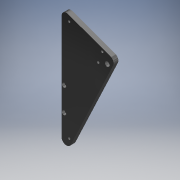
# Autodesk Inventor part: Triangle axle slide connector
Saved by Autodesk Inventor 2019 (Build 230136000, 136)
## iProperties
Part Number: Triangle axle slide connector
Material: Generic
Document SubType Name: Modeling
Designer: Delta
Appearance: Default
Author: Delta
Autodesk Inventor part; units mm, degrees
ref_plane "YZ Plane" through (0, 0, 0) normal (1, 0, 0) x (0, 1, 0)
ref_plane "XZ Plane" through (0, 0, 0) normal (0, 1, 0) x (-1, 0, 0)
ref_plane "XY Plane" through (0, 0, 0) normal (0, 0, 1) x (1, 0, 0)
sketch "Sketch1" plane through (0, 0, 0) normal (0, 0, 1) x (1, 0, 0)
  line L0 (0, 0) -> (0, 177.8)
  line L1 (0, 0) -> (53.8815, 0) construction
  line L2 (0, 177.8) -> (71.6046, 151.7381)
  line L3 (0, 177.8) -> (76.2, 177.8) construction
  line L4 (71.6046, 151.7381) -> (0, 0)
  dimension "d0" = 177.8
  dimension "d19" = 76.2
  dimension "d20" = 20
  constraints: 10 end point, 2 horizontal, 1 equal length, 1 vertical
  measures "d0" distance of L0.start L0.end
  measures "d19" distance of L0.end L2.end
  measures "d20" angle of L2 L3
extrude "Extrusion1" add sketch "Sketch1" along normal blind 6.35
fillet "Fillet1" radius 6.35 2 edges at (0, 177.8, 3.175) (0, 0, 3.175)
fillet "Fillet4" radius 6.35 1 edges at (71.6046, 151.7381, 3.175)
sketch "Sketch3" plane through (0, 0, 6.35) normal (0, 0, 1) x (1, 0, 0)
  circle A0 centre (3.175, 58.1807) radius 1.524
  circle A1 centre (3.175, 89.9307) radius 1.524
  line L0 (0, 168.7313) -> (0, 28.3357) projected
  point P0 (0, 0)
  dimension "d22" = 3.048
  dimension "d23" = 3.048
  dimension "d24" = 3.175
  dimension "d25" = 3.175
  dimension "d26" = 29.845
  dimension "d27" = 31.75
  constraints: 2 centre point
  measures "d22" diameter of A0
  measures "d23" diameter of A1
  measures "d24" distance from line of L0 A0.centre
  measures "d25" distance from line of L0 A1.centre
  measures "d26" vertical distance of L0.end A0.centre
  measures "d27" distance of A0.centre A1.centre
extrude "Extrusion3" cut sketch "Sketch3" against normal through all
sketch "Sketch4" plane through (0, 0, 6.35) normal (0, 0, 1) x (1, 0, 0)
  circle A0 centre (3.175, 58.1807) radius 1.524 projected
  circle A1 centre (3.175, 58.1807) radius 2.921
  circle A2 centre (3.175, 89.9307) radius 1.524 projected
  circle A3 centre (3.175, 89.9307) radius 2.921
  point P0 (0, 0)
  dimension "d30" = 5.842
  dimension "d31" = 5.842
  constraints: 2 centre point, 2 coincident
  measures "d30" diameter of A1
  measures "d31" diameter of A3
extrude "Extrusion4" cut sketch "Sketch4" against normal blind 3.556
sketch "Sketch5" plane through (0, 0, 6.35) normal (0, 0, 1) x (1, 0, 0)
  circle A0 centre (60.795, 143.1007) radius 3.175
  point P0 (0, 0)
  point P1 (8.5218, 174.6983)
  dimension "d34" = 6.35
  dimension "d35" = 52.2732
  dimension "d36" = 31.5976
  constraints: 1 centre point
  measures "d34" diameter of A0
  measures "d35" horizontal distance of point (8.522, 174.698) A0.centre
  measures "d36" vertical distance of A0.centre point (8.522, 174.698)
extrude "Extrusion5" cut sketch "Sketch5" against normal through all
sketch "Sketch6" plane through (0, 0, 6.35) normal (0, 0, 1) x (1, 0, 0)
  line L0 (0, 168.7313) -> (0, 28.3357) projected
  arc A0 (8.5218, 174.6983) -> (0, 168.7313) centre (6.35, 168.7313) ccw projected
  point P0 (0, 0)
  point P1 (10.0076, 166.8263)
  point P2 (10.0076, 31.8253)
  dimension "d39" = 10.0076
  dimension "d40" = 1.905
  dimension "d41" = 136.906
  dimension "d42" = 0
  measures "d39" distance from line of L0 point (10.008, 166.826)
  measures "d40" vertical distance of A0.centre point (10.008, 166.826)
  measures "d41" vertical distance of point (10.008, 31.825) A0.centre
  measures "d42" horizontal distance of point (10.008, 31.825) point (10.008, 166.826)
hole "Hole1" at (10.0076, 31.8253, 6.35) at (10.0076, 166.8263, 6.35) direction (0, 0, -1) diameter 3 end through all
sketch "Sketch7" plane through (0, 0, 6.35) normal (0, 0, 1) x (1, 0, 0)
  line L0 (65.0627, 154.1191) -> (8.5218, 174.6983) projected
  line L1 (12.0927, 25.6258) -> (68.6335, 145.4421) projected
  circle A0 centre (48.6603, 139.0056) radius 1.5875
  circle A1 centre (54.0562, 154.0707) radius 1.5875
  point P0 (0, 0)
  dimension "d52" = 3.81
  dimension "d53" = 19.812
  dimension "d54" = 15.3162
  dimension "d55" = 16.8656
  dimension "d56" = 3.175
  dimension "d57" = 3.175
  constraints: 2 centre point, 2 coincident
  measures "d52" distance from line of point (54.056, 154.071) L0
  measures "d53" distance from line of point (48.66, 139.006) L0
  measures "d54" distance from line of point (48.66, 139.006) L1
  measures "d55" distance from line of point (54.056, 154.071) L1
  measures "d56" diameter of A0
  measures "d57" diameter of A1
extrude "Extrusion6" cut sketch "Sketch7" against normal through all
equation "\"d22\" = d23"
body "Solid1"
